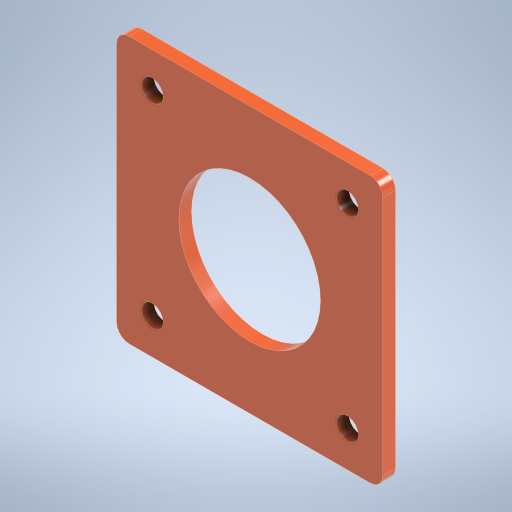
# Autodesk Inventor part: NEMA 17 Damper
Saved by Autodesk Inventor 2024 (Build 280153000, 153)
## iProperties
Created: 2024-12-26
Part Number: NEMA 17 Damper
Material: Rubber, Silicone
Document SubType Name: Modeling
Designer: Ishaan
Density: 1.25 g/cm^3
Appearance: Smooth - Light Orange
Author: Ishaan
Autodesk Inventor part; units mm, degrees
ref_plane "YZ Plane" through (0, 0, 0) normal (1, 0, 0) x (0, 1, 0)
ref_plane "XZ Plane" through (0, 0, 0) normal (0, 1, 0) x (-1, 0, 0)
ref_plane "XY Plane" through (0, 0, 0) normal (0, 0, 1) x (1, 0, 0)
sketch "Sketch1" plane through (0, 0, 0) normal (0, 0, 1) x (1, 0, 0)
  line L0 (19.15, -21.15) -> (-19.15, -21.15)
  line L1 (-21.15, -19.15) -> (-21.15, 19.15)
  line L2 (-19.15, 21.15) -> (19.15, 21.15)
  line L3 (21.15, 19.15) -> (21.15, -19.15)
  line L4 (21.15, -21.15) -> (-21.15, 21.15) construction
  line L5 (-21.15, -21.15) -> (21.15, 21.15) construction
  circle A0 centre (0, 0) radius 11.25
  line L6 (15.5, -15.5) -> (-15.5, -15.5) construction
  line L7 (-15.5, -15.5) -> (-15.5, 15.5) construction
  line L8 (-15.5, 15.5) -> (15.5, 15.5) construction
  line L9 (15.5, 15.5) -> (15.5, -15.5) construction
  line L10 (15.5, -15.5) -> (-15.5, 15.5) construction
  line L11 (-15.5, -15.5) -> (15.5, 15.5) construction
  circle A1 centre (15.5, 15.5) radius 1.75
  circle A2 centre (15.5, -15.5) radius 1.75
  circle A3 centre (-15.5, -15.5) radius 1.75
  circle A4 centre (-15.5, 15.5) radius 1.75
  arc A5 (-19.15, 21.15) -> (-21.15, 19.15) centre (-19.15, 19.15) ccw
  arc A6 (21.15, 19.15) -> (19.15, 21.15) centre (19.15, 19.15) ccw
  arc A7 (19.15, -21.15) -> (21.15, -19.15) centre (19.15, -19.15) ccw
  arc A8 (-21.15, -19.15) -> (-19.15, -21.15) centre (-19.15, -19.15) ccw
  dimension "d0" = 42.3
  dimension "d1" = 42.3
  dimension "d2" = 22.5
  dimension "d3" = 31
  dimension "d4" = 31
  dimension "d5" = 3.5
  dimension "d6" = 2
  constraints: 24 end point, 9 centre point, 8 point on circle, 8 point on line, 8 tangent, 6 equal radius, 5 coincident, 4 midpoint, 4 parallel, 2 horizontal, 2 perpendicular
  measures "d0" distance of L4.end L5.end
  measures "d1" distance of L5.start L4.end
  measures "d2" diameter of A0
  measures "d3" distance of L7.end L8.end
  measures "d4" distance of L6.end L7.end
  measures "d5" diameter of A1
  measures "d6" radius of A5
extrude "Extrusion1" add sketch "Sketch1" along normal blind 2
body "Solid1"
